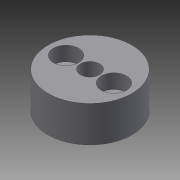
# Autodesk Inventor part: gear thrust cup
Saved by Autodesk Inventor 2014 (Build 180170000, 170)
## iProperties
Created: 2017-06-15
Part Number: gear thrust cup
Material: Generic
Document SubType Name: Modeling
Designer: RMcComber
Density: 1 g/cm^3
Appearance: Default
Author: RMcComber
Autodesk Inventor part; units mm, degrees
ref_plane "YZ Plane" through (0, 0, 0) normal (1, 0, 0) x (0, 1, 0)
ref_plane "XZ Plane" through (0, 0, 0) normal (0, 1, 0) x (-1, 0, 0)
ref_plane "XY Plane" through (0, 0, 0) normal (0, 0, 1) x (1, 0, 0)
sketch "Sketch1" plane through (0, 0, 0) normal (0, 0, 1) x (1, 0, 0)
  circle A0 centre (0, 0) radius 17.5
  circle A1 centre (0, 0) radius 4
  line L0 (-10, 0) -> (10, 0) construction
  circle A2 centre (-10, 0) radius 3
  circle A3 centre (10, 0) radius 3
  dimension "d0" = 35
  dimension "d1" = 8
  dimension "d7" = 20
  dimension "d8" = 6
  constraints: 5 coincident, 4 centre point, 2 end point, 1 equal radius, 1 horizontal, 1 midpoint
  measures "d0" diameter of A0
  measures "d1" diameter of A1
  measures "d7" distance of L0.start L0.end
  measures "d8" diameter of A2
extrude "Extrusion1" add sketch "Sketch1" along normal blind 15
sketch "Sketch3" plane through (0, 0, 15) normal (0, 0, 1) x (1, 0, 0)
  circle A0 centre (10, 0) radius 3 projected
  circle A1 centre (-10, 0) radius 3 projected
  circle A2 centre (-10, 0) radius 5.25
  circle A3 centre (10, 0) radius 5.25
  dimension "d9" = 10.5
  constraints: 2 centre point, 2 coincident, 1 equal radius
  measures "d9" diameter of A2
extrude "Extrusion3" cut sketch "Sketch3" against normal blind 6
body "Solid1"
